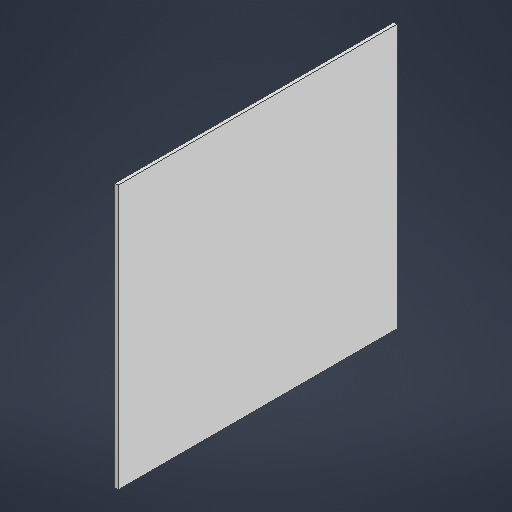
# Autodesk Inventor part: plaque_ar
Saved by Autodesk Inventor 2026 (Build 300175000, 175)
## iProperties
Created: 2025-04-19
Part Number: plaque_ar
Material: Générique
Document SubType Name: Modeling
Designer: enezl
Density: 1 g/cm^3
Appearance: Par défaut
Author: enezl
Autodesk Inventor part; units mm, degrees
ref_plane "YZ Plane" through (0, 0, 0) normal (1, 0, 0) x (0, 1, 0)
ref_plane "XZ Plane" through (0, 0, 0) normal (0, 1, 0) x (-1, 0, 0)
ref_plane "XY Plane" through (0, 0, 0) normal (0, 0, 1) x (1, 0, 0)
sketch "Esquisse1" plane through (0, 0, 0) normal (1, 0, 0) x (0, 1, 0)
  line L0 (-121, 128) -> (121, 128)
  line L1 (121, 128) -> (121, -128)
  line L2 (121, -128) -> (-121, -128)
  line L3 (-121, -128) -> (-121, 128)
  line L4 (-121, 128) -> (121, -128) construction
  line L5 (121, 128) -> (-121, -128) construction
  point P0 (0, 0)
  dimension "d0" = 256
  dimension "d1" = 242
  constraints: 12 end point, 2 midpoint, 2 parallel, 1 horizontal, 1 perpendicular
  measures "d0" distance of L0.end L1.end
  measures "d1" distance of L1.end L2.end
extrude "Extrusion1" add sketch "Esquisse1" along normal blind 3
